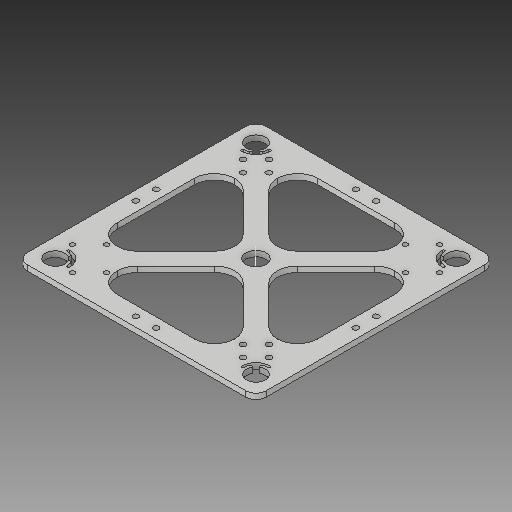
# Autodesk Inventor part: SidePanel
Saved by Autodesk Inventor 2018 (Build 220112000, 112)
## iProperties
Created: 2019-06-12
Part Number: SidePanel
Material: Generic
Document SubType Name: Modeling
Designer: anirudh
Density: 1 g/cm^3
Appearance: Default
Author: anirudh
Autodesk Inventor part; units mm, degrees
ref_plane "YZ Plane" through (0, 0, 0) normal (1, 0, 0) x (0, 1, 0)
ref_plane "XZ Plane" through (0, 0, 0) normal (0, 1, 0) x (-1, 0, 0)
ref_plane "XY Plane" through (0, 0, 0) normal (0, 0, 1) x (1, 0, 0)
sketch "Sketch1" plane through (0, 0, 0) normal (0, 1, 0) x (-1, 0, 0)
  line L0 (0, 0) -> (150, 0)
  line L1 (150, 0) -> (150, -150)
  line L2 (150, -150) -> (0, -150)
  line L3 (0, -150) -> (0, 0)
  line L4 (150, 0) -> (150, -30)
  line L5 (150, 0) -> (150, -24)
  arc A0 (135.0185, -17.2068) -> (132.7932, -14.9815) centre (138, -12) ccw
  line L6 (150, 0) -> (111.9, 0)
  line L7 (150, -38.1) -> (150, 0)
  line L8 (150, 0) -> (111.9, 0)
  line L9 (111.9, -12) -> (111.9, -30.0178)
  line L10 (119.9822, -38.1) -> (138, -38.1)
  line L11 (150, -38.1) -> (150, 0)
  line L12 (79.6178, -62.3) -> (70.3822, -62.3)
  line L13 (62.3, -70.3822) -> (62.3, -79.6178)
  line L14 (70.3822, -87.7) -> (79.6178, -87.7)
  line L15 (87.7, -79.6178) -> (87.7, -70.3822)
  line L16 (111.9, -138) -> (111.9, -119.9822)
  line L17 (119.9822, -111.9) -> (138, -111.9)
  line L18 (38.1, -12) -> (38.1, -30.0178)
  line L19 (30.0178, -38.1) -> (12, -38.1)
  line L20 (38.1, -138) -> (38.1, -119.9822)
  line L21 (30.0178, -111.9) -> (12, -111.9)
  line L22 (111.9, -12) -> (38.1, -12)
  line L23 (138, -38.1) -> (138, -111.9)
  line L24 (111.9, -138) -> (38.1, -138)
  line L25 (12, -111.9) -> (12, -38.1)
  line L26 (119.9822, -38.1) -> (128.6968, -38.1) construction
  line L27 (119.9822, -111.9) -> (124.7995, -111.9) construction
  line L28 (38.1, -38.1) -> (54.2899, -38.1) construction
  line L29 (38.1, -111.9) -> (59.1951, -111.9) construction
  line L30 (101.8805, -40.0373) -> (111.9, -30.0178)
  line L31 (105.4618, -52.6204) -> (119.9822, -38.1)
  line L32 (105.9614, -97.8792) -> (119.9822, -111.9)
  line L33 (99.7767, -107.8589) -> (111.9, -119.9822)
  line L34 (49.2133, -41.1311) -> (38.1, -30.0178)
  line L35 (42.9525, -51.0347) -> (30.0178, -38.1)
  line L36 (41.1728, -100.745) -> (30.0178, -111.9)
  line L37 (51.8972, -106.185) -> (38.1, -119.9822)
  line L38 (87.7, -70.3822) -> (115.9411, -42.1411)
  line L39 (115.9411, -107.8589) -> (87.7, -79.6178)
  line L40 (107.8589, -34.0589) -> (79.6178, -62.3)
  line L41 (70.3822, -62.3) -> (42.1411, -34.0589)
  line L42 (34.0589, -42.1411) -> (62.3, -70.3822)
  line L43 (62.3, -79.6178) -> (34.0589, -107.8589)
  line L44 (42.1411, -115.9411) -> (70.3822, -87.7)
  line L45 (79.6178, -87.7) -> (107.8589, -115.9411)
  arc A1 (128.825, -12) -> (138, -21.175) centre (138, -12) ccw
  arc A2 (130.4125, -12) -> (128.825, -12) centre (129.6188, -12) ccw
  arc A3 (138, -21.175) -> (138, -19.5875) centre (138, -20.3813) ccw
  arc A4 (131.0884, -15.1305) -> (132.7932, -14.9815) centre (131.851, -14.0291) ccw
  arc A5 (135.0185, -17.2068) -> (134.8695, -18.9116) centre (135.9709, -18.149) ccw
  arc A6 (130.4125, -12) -> (131.0884, -15.1305) centre (138, -12) ccw
  arc A7 (134.8695, -18.9116) -> (138, -19.5875) centre (138, -12) ccw
  arc A8 (132.7932, -135.0185) -> (135.0185, -132.7932) centre (138, -138) ccw
  arc A9 (138, -128.825) -> (128.825, -138) centre (138, -138) ccw
  arc A10 (128.825, -138) -> (130.4125, -138) centre (129.6188, -138) ccw
  arc A11 (138, -130.4125) -> (138, -128.825) centre (138, -129.6187) ccw
  arc A12 (132.7932, -135.0185) -> (131.0884, -134.8695) centre (131.851, -135.9709) ccw
  arc A13 (134.8695, -131.0884) -> (135.0185, -132.7932) centre (135.9709, -131.851) ccw
  arc A14 (131.0884, -134.8695) -> (130.4125, -138) centre (138, -138) ccw
  arc A15 (138, -130.4125) -> (134.8695, -131.0884) centre (138, -138) ccw
  arc A16 (17.2068, -14.9815) -> (14.9815, -17.2068) centre (12, -12) ccw
  arc A17 (12, -21.175) -> (21.175, -12) centre (12, -12) ccw
  arc A18 (21.175, -12) -> (19.5875, -12) centre (20.3812, -12) ccw
  arc A19 (12, -19.5875) -> (12, -21.175) centre (12, -20.3813) ccw
  arc A20 (17.2068, -14.9815) -> (18.9116, -15.1305) centre (18.149, -14.0291) ccw
  arc A21 (15.1305, -18.9116) -> (14.9815, -17.2068) centre (14.0291, -18.149) ccw
  arc A22 (18.9116, -15.1305) -> (19.5875, -12) centre (12, -12) ccw
  arc A23 (12, -19.5875) -> (15.1305, -18.9116) centre (12, -12) ccw
  arc A24 (19.5875, -138) -> (18.9116, -134.8695) centre (12, -138) ccw
  arc A25 (19.5875, -138) -> (21.175, -138) centre (20.3812, -138) ccw
  arc A26 (15.1305, -131.0884) -> (12, -130.4125) centre (12, -138) ccw
  arc A27 (21.175, -138) -> (12, -128.825) centre (12, -138) ccw
  arc A28 (12, -128.825) -> (12, -130.4125) centre (12, -129.6187) ccw
  arc A29 (14.9815, -132.7932) -> (17.2068, -135.0185) centre (12, -138) ccw
  arc A30 (18.9116, -134.8695) -> (17.2068, -135.0185) centre (18.149, -135.9709) ccw
  arc A31 (14.9815, -132.7932) -> (15.1305, -131.0884) centre (14.0291, -131.851) ccw
  dimension "d0" = 150
  constraints: 92 end point, 64 point on circle, 32 centre point, 10 point on line, 8 coincident, 8 horizontal, 7 perpendicular, 6 parallel
  measures "d0" distance of L1.end L2.end
extrude "Extrusion2" add sketch "Sketch1" along normal blind 3.5
fillet "Fillet1" radius 6.35 4 edges at (-150, 1.75, 0) (0, 1.75, 0) (0, 1.75, -150) (-150, 1.75, -150)
fillet "Fillet2" radius 12.7 24 edges at (-111.9, 1.75, -30.0178) (-111.9, 1.75, -12) (-79.6178, 1.75, -62.3) (-70.3822, 1.75, -62.3) (-38.1, 1.75, -12) (-38.1, 1.75, -30.0178) (-87.7, 1.75, -79.6178) (-119.9822, 1.75, -111.9) (-138, 1.75, -111.9) (-138, 1.75, -38.1) (-119.9822, 1.75, -38.1) (-87.7, 1.75, -70.3822) (-79.6178, 1.75, -87.7) (-70.3822, 1.75, -87.7) (-111.9, 1.75, -119.9822) (-111.9, 1.75, -138) (-38.1, 1.75, -138) (-38.1, 1.75, -119.9822) (-12, 1.75, -38.1) (-12, 1.75, -111.9) (-30.0178, 1.75, -111.9) (-62.3, 1.75, -79.6178) (-62.3, 1.75, -70.3822) (-30.0178, 1.75, -38.1)
sketch "Sketch2" plane through (0, 3.5, 0) normal (0, 1, 0) x (1, 0, 0)
  arc A0 (-150, 6.35) -> (-143.65, 0) centre (-143.65, 6.35) ccw projected
  arc A1 (0, 143.65) -> (-6.35, 150) centre (-6.35, 143.65) ccw projected
  arc A2 (-111.9, 24.7) -> (-99.2, 12) centre (-99.2, 24.7) ccw projected
  arc A3 (-138, 50.8) -> (-125.3, 38.1) centre (-125.3, 50.8) ccw projected
  arc A4 (-128.825, 12) -> (-138, 21.175) centre (-138, 12) ccw projected
  circle A5 centre (-124.7485, 17.112) radius 1.8
  circle A6 centre (-117.5643, 24.2962) radius 1.8
  circle A7 centre (-132.888, 25.2515) radius 1.8
  circle A8 centre (-125.7038, 32.4357) radius 1.8
  arc A9 (-132.7932, 135.0185) -> (-135.0185, 132.7932) centre (-138, 138) ccw projected
  line L0 (-150, 143.65) -> (-150, 6.35) projected
  circle A10 centre (-144, 68.65) radius 1.8
  line L1 (-50.8, 12) -> (-99.2, 12) projected
  circle A11 centre (-81.35, 6) radius 1.8
  circle A12 centre (-124.7485, 132.888) radius 1.8
  circle A13 centre (-117.5643, 125.7038) radius 1.8
  circle A14 centre (-132.888, 124.7485) radius 1.8
  circle A15 centre (-125.7038, 117.5643) radius 1.8
  circle A16 centre (-144, 81.35) radius 1.8
  circle A17 centre (-81.35, 144) radius 1.8
  circle A18 centre (-25.2515, 17.112) radius 1.8
  circle A19 centre (-32.4357, 24.2962) radius 1.8
  circle A20 centre (-17.112, 25.2515) radius 1.8
  circle A21 centre (-24.2962, 32.4357) radius 1.8
  circle A22 centre (-6, 68.65) radius 1.8
  circle A23 centre (-68.65, 6) radius 1.8
  circle A24 centre (-68.65, 144) radius 1.8
  circle A25 centre (-32.4357, 125.7038) radius 1.8
  circle A26 centre (-25.2515, 132.888) radius 1.8
  circle A27 centre (-24.2962, 117.5643) radius 1.8
  circle A28 centre (-17.112, 124.7485) radius 1.8
  circle A29 centre (-6, 81.35) radius 1.8
  point P0 (0, 0)
  point P1 (-6.35, 0)
  dimension "d42" = 3.6
  dimension "d44" = 3.6
  dimension "d45" = 3.6
  dimension "d46" = 3.6
  dimension "d50" = 3.6
  dimension "d53" = 3.6
  constraints: 24 centre point
  measures "d42" diameter of A5
  measures "d44" diameter of A6
  measures "d45" diameter of A7
  measures "d46" diameter of A8
  measures "d50" diameter of A10
  measures "d53" diameter of A11
extrude "Extrusion3" cut sketch "Sketch2" against normal blind 3.5
ref_plane "Work Plane1" through (-6.35, 0, -75) normal (0, 0, -1) x (-1, 0, 0)
ref_plane "Work Plane2" through (-75, 0, -143.65) normal (-1, 0, 0) x (0, 0, 1)
sketch "Sketch4" plane through (0, 3.5, 0) normal (0, 1, 0) x (1, 0, 0)
  arc A0 (-116.2625, 108.1803) -> (-125.2427, 111.9) centre (-125.2427, 99.2) ccw projected
  arc A1 (-116.2625, 108.1803) -> (-125.2427, 111.9) centre (-125.2427, 99.2) ccw
  arc A2 (-111.9, 125.2427) -> (-108.1803, 116.2625) centre (-99.2, 125.2427) ccw projected
  arc A3 (-111.9, 125.2427) -> (-108.1803, 116.2625) centre (-99.2, 125.2427) ccw
  line L0 (-108.1803, 116.2625) -> (-83.9803, 92.0625) projected
  line L1 (-116.2625, 108.1803) -> (-108.1803, 116.2625)
  line L2 (-125.2427, 111.9) -> (-139.71, 126.3673)
  line L3 (-111.9, 125.2427) -> (-125.8843, 139.227)
  arc A4 (-137.219, 128.8583) -> (-128.8583, 137.219) centre (-138, 138) ccw
  line L4 (-126.3673, 139.71) -> (-125.8843, 139.227)
  line L5 (-139.71, 126.3673) -> (-137.219, 128.8583)
  line L6 (-128.8583, 137.219) -> (-126.3673, 139.71)
  circle A5 centre (-132.888, 124.7485) radius 1.8 projected
  circle A6 centre (-132.888, 124.7485) radius 1.8
  circle A7 centre (-125.7038, 117.5643) radius 1.8 projected
  circle A8 centre (-125.7038, 117.5643) radius 1.8
  circle A9 centre (-124.7485, 132.888) radius 1.8 projected
  circle A10 centre (-124.7485, 132.888) radius 1.8
  circle A11 centre (-117.5643, 125.7038) radius 1.8 projected
  circle A12 centre (-117.5643, 125.7038) radius 1.8
  point P0 (0, 0)
  point P1 (-138, 128.825)
  constraints: 12 end point, 7 centre point, 7 point on circle, 5 coincident, 1 collinear, 1 perpendicular
sketch "Sketch5" plane through (0, 3.5, 0) normal (0, 1, 0) x (1, 0, 0)
  arc A0 (-83.9803, 92.0625) -> (-66.0197, 92.0625) centre (-75, 101.0427) ccw projected
  arc A1 (-66.0197, 57.9375) -> (-83.9803, 57.9375) centre (-75, 48.9573) ccw projected
  arc A2 (-57.9375, 83.9803) -> (-57.9375, 66.0197) centre (-48.9573, 75) ccw projected
  arc A3 (-92.0625, 66.0197) -> (-92.0625, 83.9803) centre (-101.0427, 75) ccw projected
  circle A4 centre (-75, 75) radius 6.35
  point P0 (0, 0)
  dimension "d56" = 12.7
  constraints: 1 centre point
  measures "d56" diameter of A4
extrude "Extrusion4" cut sketch "Sketch5" against normal blind 25.4
sketch "Sketch6" plane through (0, 3.5, 0) normal (0, 1, 0) x (1, 0, 0)
  circle A0 centre (-17.112, 124.7485) radius 1.8 projected
  circle A1 centre (-17.112, 124.7485) radius 1.8
  circle A2 centre (-24.2962, 117.5643) radius 1.8 projected
  circle A3 centre (-24.2962, 117.5643) radius 1.8
  circle A4 centre (-25.2515, 132.888) radius 1.8 projected
  circle A5 centre (-25.2515, 132.888) radius 1.8
  circle A6 centre (-32.4357, 125.7038) radius 1.8 projected
  circle A7 centre (-32.4357, 125.7038) radius 1.8
  circle A8 centre (-117.5643, 24.2962) radius 1.8 projected
  circle A9 centre (-117.5643, 24.2962) radius 1.8
  circle A10 centre (-124.7485, 17.112) radius 1.8 projected
  circle A11 centre (-124.7485, 17.112) radius 1.8
  circle A12 centre (-125.7038, 32.4357) radius 1.8 projected
  circle A13 centre (-125.7038, 32.4357) radius 1.8
  circle A14 centre (-132.888, 25.2515) radius 1.8 projected
  circle A15 centre (-132.888, 25.2515) radius 1.8
  constraints: 8 centre point, 8 coincident
extrude "Extrusion5" add sketch "Sketch6" against normal blind 3.5
sketch "Sketch7" plane through (0, 3.5, 0) normal (0, 1, 0) x (1, 0, 0)
  circle A0 centre (-114.2023, 20.5312) radius 1.5
  circle A1 centre (-129.4688, 35.7977) radius 1.5
  circle A2 centre (-140.2451, 25.0214) radius 1.5
  circle A3 centre (-124.9786, 9.7549) radius 1.5
  circle A4 centre (-20.5312, 114.2023) radius 1.5
  circle A5 centre (-35.7977, 129.4688) radius 1.5
  circle A6 centre (-25.0214, 140.2451) radius 1.5
  circle A7 centre (-9.7549, 124.9786) radius 1.5
  arc A8 (-135.0185, 17.2068) -> (-132.7932, 14.9815) centre (-138, 12) ccw projected
  line L0 (-138, 12) -> (-122.76, 12) construction
  arc A9 (-14.9815, 132.7932) -> (-17.2068, 135.0185) centre (-12, 138) ccw projected
  line L1 (-12, 138) -> (3.24, 138) construction
  dimension "d66" = 3
  dimension "d67" = 3
  dimension "d68" = 3
  dimension "d69" = 3
  constraints: 8 centre point, 4 end point, 2 horizontal
  measures "d66" diameter of A0
  measures "d67" diameter of A1
  measures "d68" diameter of A2
  measures "d69" diameter of A3
extrude "Extrusion7" cut sketch "Sketch7" against normal blind 6.35
sketch "Sketch9" plane through (0, 3.5, 0) normal (0, 1, 0) x (1, 0, 0)
  arc A0 (-17.2068, 14.9815) -> (-14.9815, 17.2068) centre (-12, 12) ccw projected
  arc A1 (-17.2068, 14.9815) -> (-14.9815, 17.2068) centre (-12, 12) ccw
  arc A2 (-17.2068, 14.9815) -> (-18.9116, 15.1305) centre (-18.149, 14.0291) ccw projected
  arc A3 (-17.2068, 14.9815) -> (-18.9116, 15.1305) centre (-18.149, 14.0291) ccw
  arc A4 (-15.1305, 18.9116) -> (-14.9815, 17.2068) centre (-14.0291, 18.149) ccw projected
  arc A5 (-15.1305, 18.9116) -> (-14.9815, 17.2068) centre (-14.0291, 18.149) ccw
  arc A6 (-12, 19.5875) -> (-15.1305, 18.9116) centre (-12, 12) ccw projected
  arc A7 (-12, 21.175) -> (-21.175, 12) centre (-12, 12) ccw projected
  arc A8 (-12, 21.175) -> (-21.175, 12) centre (-12, 12) ccw
  arc A9 (-21.175, 12) -> (-19.5875, 12) centre (-20.3812, 12) ccw projected
  arc A10 (-21.175, 12) -> (-19.5875, 12) centre (-20.3812, 12) ccw
  arc A11 (-12, 19.5875) -> (-12, 21.175) centre (-12, 20.3813) ccw projected
  arc A12 (-12, 19.5875) -> (-12, 21.175) centre (-12, 20.3813) ccw
  arc A13 (-12, 19.5875) -> (-15.1305, 18.9116) centre (-12, 12) ccw
  arc A14 (-18.9116, 15.1305) -> (-19.5875, 12) centre (-12, 12) ccw
  point P0 (0, 0)
  constraints: 18 point on circle, 8 centre point, 7 coincident
body "Solid2"
